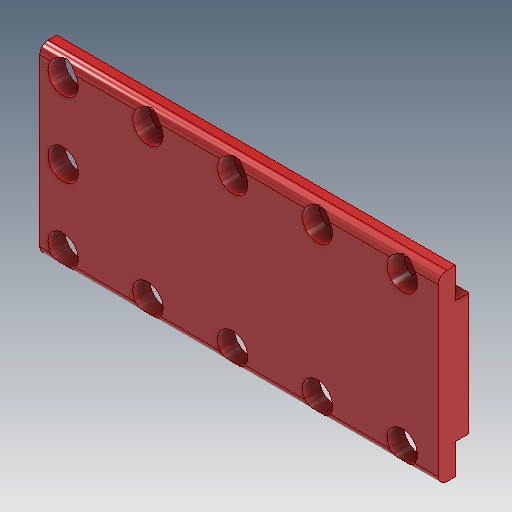
# Autodesk Inventor part: Cover part of robot arm bottom side
Saved by Autodesk Inventor 2020.3 (Build 243373010, 373A)
## iProperties
Created: 2021-04-24
Part Number: Cover part of robot arm bottom side
Material: Steel, Alloy
Document SubType Name: Modeling
Designer: marti
Density: 7.73 g/cm^3
Appearance: Red
Mass: 2860.3 g
Surface Area: 619.586 cm^2
Volume: 370.025 cm^3
Author: marti
Autodesk Inventor part; units mm, degrees
ref_plane "YZ Plane" through (0, 0, 0) normal (1, 0, 0) x (0, 1, 0)
ref_plane "XZ Plane" through (0, 0, 0) normal (0, 1, 0) x (-1, 0, 0)
ref_plane "XY Plane" through (0, 0, 0) normal (0, 0, 1) x (1, 0, 0)
sketch "Sketch1" plane through (0, 0, 0) normal (0, 0, 1) x (1, 0, 0)
  line L0 (-117.5, 54) -> (117.5, 54)
  line L1 (117.5, 54) -> (117.5, -54)
  line L2 (117.5, -54) -> (-117.5, -54)
  line L3 (-117.5, -54) -> (-117.5, 54)
  line L4 (-88.19, 36) -> (117.5, 36)
  line L5 (117.5, 36) -> (117.5, -36)
  line L6 (117.5, -36) -> (-88.19, -36)
  line L7 (-88.19, -36) -> (-88.19, 36)
  point P0 (0, 0)
  point P1 (117.5, 0)
  point P2 (0, 54)
  point P3 (117.5, 0)
  point P4 (117.5, -36)
  dimension "d0" = 108
  dimension "d1" = 235
  dimension "d4" = 205.69
  dimension "d5" = 72
  constraints: 16 end point, 4 parallel, 3 midpoint, 2 coincident, 2 horizontal, 2 perpendicular, 1 horizontal alignment, 1 vertical alignment
  measures "d0" distance of L0.end L1.end
  measures "d1" distance of L0.start L0.end
  measures "d4" distance of L5.end L6.end
  measures "d5" distance of L4.end L5.end
extrude "Extrusion2" add sketch "Sketch1" against normal blind 10 contours L1 L6 L7 L4
extrude "Extrusion3" add sketch "Sketch1" along normal blind 10
chamfer "Chamfer1" distance 2 angle 45 4 edges at (14.655, -36, -10) (14.655, 36, -10) (-88.19, 0, -10) (117.5, 0, -10)
fillet "Fillet1" radius 5 2 edges at (0, 54, 10) (0, -54, 10)
sketch "Sketch3" plane through (0, 0, 10) normal (0, 0, 1) x (1, 0, 0)
  line L0 (117.5, -49) -> (-117.5, -49) projected
  line L1 (-117.5, 49) -> (117.5, 49) projected
  line L2 (-117.5, -54) -> (117.5, -54) projected
  line L3 (117.5, 54) -> (-117.5, 54) projected
  line L4 (-117.5, 49) -> (-117.5, -49) projected
  line L5 (117.5, -49) -> (117.5, 49) projected
  point P0 (-103.7107, 43.9255)
  point P1 (-103.7107, 0)
  point P2 (-103.7107, -43.9255)
  point P3 (-117.5, 0)
  dimension "d18" = 98
  dimension "d19" = 108
  dimension "d20" = 87.851
  dimension "d21" = 43.9255
  dimension "d22" = 221.2107
  constraints: 2 vertical alignment, 1 horizontal alignment, 1 midpoint
  measures "d18" distance between parallel lines of L0 L1
  measures "d19" distance between parallel lines of L2 L3
  measures "d20" distance of point (-103.711, -43.925) point (-103.711, 43.925)
  measures "d21" distance of point (-103.711, 43.925) point (-103.711, 0)
  measures "d22" distance from line of L5 point (-103.711, 43.925)
hole "Hole1" at (-103.7107, 43.9255, 10) at (-103.7107, -43.9255, 10) direction (0, 0, -1) diameter 18 depth 50 tip angle 118
pattern_linear "Rectangular Pattern1" count 5 spacing 50 along (1, 0, 0) of "Hole1"
hole "Hole2" at (-103.7107, 0, 10) direction (0, 0, -1) diameter 18 depth 15 tip angle 118
equation "\"d21\" = 0.5 * d20"
body "Solid2"
